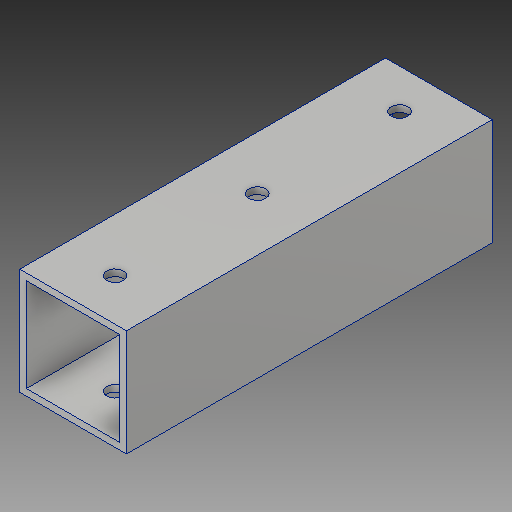
# Autodesk Inventor part: ST01
Saved by Autodesk Inventor 2017 (Build 210142000, 142)
## iProperties
Created: 2019-05-24
Part Number: ST01
Material: Aluminum 6061
Document SubType Name: Modeling
Designer: Dell
Density: 2.7 g/cm^3
Appearance: Aluminum - Flat
Mass: 281.812 g
Surface Area: 674.364 cm^2
Volume: 104.375 cm^3
Author: Dell
Autodesk Inventor part; units mm, degrees
ref_plane "YZ Plane" through (0, 0, 0) normal (1, 0, 0) x (0, 1, 0)
ref_plane "XZ Plane" through (0, 0, 0) normal (0, 1, 0) x (-1, 0, 0)
ref_plane "XY Plane" through (0, 0, 0) normal (0, 0, 1) x (1, 0, 0)
sketch "Sketch1" plane through (0, 0, 0) normal (0, 0, 1) x (1, 0, 0)
  line L0 (0, 0) -> (50.8, 0)
  line L1 (50.8, 0) -> (50.8, 50.8)
  line L2 (50.8, 50.8) -> (0, 50.8)
  line L3 (0, 50.8) -> (0, 0)
  line L4 (3.175, 3.175) -> (47.625, 3.175)
  line L5 (47.625, 3.175) -> (47.625, 47.625)
  line L6 (47.625, 47.625) -> (3.175, 47.625)
  line L7 (3.175, 47.625) -> (3.175, 3.175)
  dimension "d0" = 50.8
  dimension "d1" = 50.8
  dimension "d2" = 3.175
  constraints: 16 end point, 4 parallel, 2 perpendicular, 1 horizontal, 3 other
  measures "d0" distance of L2.end L1.end
  measures "d1" distance of L1.end L0.end
  measures "d2" distance between parallel lines of L3 L7
extrude "Extrusion1" add sketch "Sketch1" along normal blind 263.05
sketch "Sketch2" plane through (0, 0, 0) normal (0, -1, 0) x (1, 0, 0)
  circle A0 centre (25.4, 107.63) radius 4
  line L0 (0, 0) -> (50.8, 0) projected
  circle A1 centre (25.4, 175.34) radius 4
  circle A2 centre (25.4, 243.05) radius 4
  point P0 (25.4, 0)
  dimension "d5" = 8
  dimension "d6" = 107.63
  dimension "d7" = 8
  dimension "d8" = 8
  dimension "d9" = 67.71
  dimension "d10" = 67.71
  constraints: 3 centre point, 3 vertical alignment, 1 midpoint
  measures "d5" diameter of A0
  measures "d6" distance from line of L0 A0.centre
  measures "d7" diameter of A1
  measures "d8" diameter of A2
  measures "d9" distance of A0.centre A1.centre
  measures "d10" distance of A1.centre A2.centre
extrude "Extrusion2" cut sketch "Sketch2" against normal through all
sketch "Sketch3" plane through (0, 0, 0) normal (0, -1, 0) x (1, 0, 0)
  line L0 (50.8, 0) -> (50.8, 263.05) projected
  line L1 (0, 0) -> (50.8, 0)
  line L2 (50.8, 0) -> (50.8, 88.9)
  line L3 (50.8, 88.9) -> (0, 88.9)
  line L4 (0, 88.9) -> (0, 0)
  dimension "d13" = 88.9
  constraints: 8 end point, 2 parallel, 1 horizontal, 1 perpendicular, 1 point on line
  measures "d13" distance between parallel lines of L1 L3
extrude "Extrusion3" cut sketch "Sketch3" against normal through all
body "Solid1"
